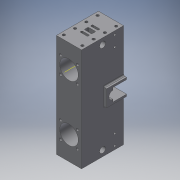
# Autodesk Inventor part: Carcassa
Saved by Autodesk Inventor 2016 (Build 200138000, 138)
## iProperties
Created: 2016-10-26
Part Number: Carcassa
Material: Generic
Document SubType Name: Modeling
Designer: 602199
Density: 1 g/cm^3
Appearance: Default
Author: 602199
Autodesk Inventor part; units mm, degrees
sketch "Sketch1" plane through (0, 0, 0) normal (0, 1, 0) x (-1, 0, 0)
  line L0 (-19, 77.75) -> (19, 77.75)
  line L1 (19, 77.75) -> (19, -77.75)
  line L2 (19, -77.75) -> (-19, -77.75)
  line L3 (-19, -77.75) -> (-19, 77.75)
  line L4 (-19, 77.75) -> (19, -77.75) construction
  line L5 (19, 77.75) -> (-19, -77.75) construction
  point P0 (0, 0)
  dimension "d0" = 38
  dimension "d1" = 155.5
  constraints: 12 end point, 2 midpoint, 2 parallel, 1 horizontal, 1 perpendicular
  measures "d0" distance of L1.end L2.end
  measures "d1" distance of L0.end L1.end
extrude "Extrusion1" add sketch "Sketch1" along normal blind 63.5
sketch "Sketch2" plane through (0, 0, 0) normal (1, 0, 0) x (0, 1, 0)
  line L0 (63.5, 77.75) -> (63.5, -77.75) construction
  line L1 (63.5, 0) -> (33.5, 0) construction
  line L2 (63.5, 0) -> (63.5, 12.5) construction
  line L3 (63.5, 12.5) -> (33.5, 12.5)
  line L4 (33.5, 12.5) -> (33.5, -12.5)
  line L5 (33.5, -12.5) -> (63.5, -12.5)
  line L6 (63.5, -12.5) -> (63.5, 12.5)
  point P0 (0, 0)
  dimension "d6" = 25
  constraints: 12 end point, 2 horizontal, 2 parallel, 1 midpoint, 1 perpendicular, 1 point on line
  measures "d6" distance of L4.end L3.end
extrude "Extrusion2" add sketch "Sketch2" along normal mid plane 47
sketch "Sketch3" plane through (0, 0, 0) normal (1, 0, 0) x (0, 1, 0)
  line L0 (63.5, 12.5) -> (63.5, -12.5) construction
  line L1 (63.5, 0) -> (42.8, 0) construction
  line L2 (63.5, 0) -> (63.5, 9.5) construction
  line L3 (63.5, 9.5) -> (42.8, 9.5)
  line L4 (42.8, 9.5) -> (42.8, -9.5)
  line L5 (42.8, -9.5) -> (63.5, -9.5)
  line L6 (63.5, -9.5) -> (63.5, 9.5)
  point P0 (0, 0)
  dimension "d9" = 20.7
  dimension "d11" = 9.5
  dimension "d12" = 19
  constraints: 12 end point, 2 horizontal, 2 parallel, 1 midpoint, 1 perpendicular, 1 point on line
  measures "d9" distance of L1.start L1.end
  measures "d11" distance of L1.start L2.end
  measures "d12" distance of L4.end L3.end
extrude "Extrusion3" cut sketch "Sketch3" along normal through all both and the other way through all
sketch "Sketch4" plane through (0, 0, 0) normal (1, 0, 0) x (0, 1, 0)
  line L0 (42.8, 9.5) -> (42.8, -9.5) projected
  circle A0 centre (42.8, 0) radius 6
  point P0 (0, 0)
  dimension "d15" = 12
  constraints: 1 centre point, 1 midpoint
  measures "d15" diameter of A0
extrude "Extrusion4" cut sketch "Sketch4" along normal through all both and the other way through all
sketch "Sketch5" plane through (19, 0, -77.75) normal (0, 0, -1) x (-1, 0, 0)
  line L0 (19, 0) -> (19, 63.5) construction
  line L1 (0, 63.5) -> (38, 63.5) construction
  line L2 (5, 6.25) -> (33, 6.25) construction
  line L3 (33, 6.25) -> (33, 57.25) construction
  line L4 (33, 57.25) -> (5, 57.25) construction
  line L5 (5, 57.25) -> (5, 6.25) construction
  line L6 (5, 6.25) -> (33, 57.25) construction
  line L7 (33, 6.25) -> (5, 57.25) construction
  circle A0 centre (5, 57.25) radius 2
  circle A1 centre (5, 6.25) radius 2
  circle A2 centre (33, 6.25) radius 2
  circle A3 centre (33, 57.25) radius 2
  line L8 (19, 31.75) -> (19, 40.25) construction
  line L9 (19, 40.25) -> (19, 23.25) construction
  circle A4 centre (5, 40.25) radius 2
  circle A5 centre (5, 23.25) radius 2
  circle A6 centre (33, 40.25) radius 2
  circle A7 centre (33, 23.25) radius 2
  dimension "d18" = 28
  dimension "d19" = 51
  dimension "d20" = 4
  dimension "d21" = 4
  dimension "d22" = 8.5
  dimension "d23" = 17
  constraints: 18 end point, 8 centre point, 6 point on line, 4 coincident, 4 midpoint, 2 parallel, 1 horizontal, 1 perpendicular
  measures "d18" distance of L4.end L3.end
  measures "d19" distance of L3.end L2.end
  measures "d20" diameter of A0
  measures "d21" diameter of A2
  measures "d22" distance of L8.start L8.end
  measures "d23" distance of L8.end L9.end
hole "Hole1" at (14, 57.25, -77.75) at (14, 40.25, -77.75) at (14, 23.25, -77.75) at (14, 6.25, -77.75) at (-14, 57.25, -77.75) at (-14, 40.25, -77.75) at (-14, 23.25, -77.75) at (-14, 6.25, -77.75) direction (0, 0, 1) diameter 4 depth 8
sketch "Sketch6" plane through (19, 0, -77.75) normal (0, 0, -1) x (-1, 0, 0)
  line L0 (19, 0) -> (19, 63.5) construction
  line L1 (0, 63.5) -> (38, 63.5) construction
  line L2 (5, 6.25) -> (33, 6.25) construction
  line L3 (33, 6.25) -> (33, 57.25) construction
  line L4 (33, 57.25) -> (5, 57.25) construction
  line L5 (5, 57.25) -> (5, 6.25) construction
  line L6 (5, 6.25) -> (33, 57.25) construction
  line L7 (33, 6.25) -> (5, 57.25) construction
  circle A0 centre (5, 57.25) radius 2
  circle A1 centre (5, 6.25) radius 2
  circle A2 centre (33, 6.25) radius 2
  circle A3 centre (33, 57.25) radius 2
  line L8 (19, 31.75) -> (19, 40.25) construction
  line L9 (19, 40.25) -> (19, 23.25) construction
  circle A4 centre (5, 40.25) radius 2
  circle A5 centre (5, 23.25) radius 2
  circle A6 centre (33, 40.25) radius 2
  circle A7 centre (33, 23.25) radius 2
  dimension "d31" = 28
  dimension "d32" = 51
  dimension "d33" = 4
  dimension "d34" = 4
  dimension "d35" = 8.5
  dimension "d36" = 17
  constraints: 20 end point, 8 centre point, 6 point on line, 4 coincident, 4 midpoint, 2 parallel, 1 horizontal, 1 perpendicular
  measures "d31" distance of L5.start L3.end
  measures "d32" distance of L3.end L3.start
  measures "d33" diameter of A0
  measures "d34" diameter of A2
  measures "d35" distance of L8.start L8.end
  measures "d36" distance of L8.end L9.end
hole "Hole2" at (14, 57.25, -77.75) at (-14, 57.25, -77.75) at (14, 40.25, -77.75) at (-14, 40.25, -77.75) at (-14, 23.25, -77.75) at (14, 23.25, -77.75) at (14, 6.25, -77.75) at (-14, 6.25, -77.75) direction (0, 0, 1) diameter 3.5 depth 12 tip angle 118
sketch "Sketch7" plane through (19, 0, -77.75) normal (0, 0, -1) x (-1, 0, 0)
  line L0 (0, 63.5) -> (38, 63.5) construction
  line L1 (19, 63.5) -> (19, 0) construction
  line L2 (19, 31.75) -> (38, 31.75) construction
  line L3 (13.25, 28.65) -> (24.75, 28.65)
  line L4 (24.75, 28.65) -> (24.75, 34.85)
  line L5 (24.75, 34.85) -> (13.25, 34.85)
  line L6 (13.25, 34.85) -> (13.25, 28.65)
  line L7 (13.25, 28.65) -> (24.75, 34.85) construction
  line L8 (24.75, 28.65) -> (13.25, 34.85) construction
  line L9 (19, 31.75) -> (19, 39.675) construction
  line L10 (19, 39.675) -> (19, 23.825) construction
  line L11 (13.25, 41.275) -> (24.75, 41.275)
  line L12 (24.75, 41.275) -> (24.75, 38.075)
  line L13 (24.75, 38.075) -> (13.25, 38.075)
  line L14 (13.25, 38.075) -> (13.25, 41.275)
  line L15 (13.25, 41.275) -> (24.75, 38.075) construction
  line L16 (24.75, 41.275) -> (13.25, 38.075) construction
  line L17 (13.25, 25.425) -> (24.75, 25.425)
  line L18 (24.75, 25.425) -> (24.75, 22.225)
  line L19 (24.75, 22.225) -> (13.25, 22.225)
  line L20 (13.25, 22.225) -> (13.25, 25.425)
  line L21 (13.25, 25.425) -> (24.75, 22.225) construction
  line L22 (24.75, 25.425) -> (13.25, 22.225) construction
  dimension "d44" = 11.5
  dimension "d45" = 6.2
  dimension "d46" = 7.925
  dimension "d47" = 15.85
  dimension "d48" = 11.5
  dimension "d49" = 3.2
  dimension "d50" = 3.2
  constraints: 44 end point, 8 midpoint, 6 parallel, 4 horizontal, 3 perpendicular, 3 point on line, 1 vertical
  measures "d44" distance of L5.end L4.end
  measures "d45" distance of L4.end L3.end
  measures "d46" distance of L2.start L9.end
  measures "d47" distance of L9.end L10.end
  measures "d48" distance of L12.end L13.end
  measures "d49" distance of L11.end L12.end
  measures "d50" distance of L17.end L18.end
extrude "Extrusion5" cut sketch "Sketch7" against normal blind 9
fillet "Fillet1" radius 1 12 edges at (5.75, 41.275, -73.25) (5.75, 38.075, -73.25) (5.75, 34.85, -73.25) (5.75, 28.65, -73.25) (5.75, 25.425, -73.25) (5.75, 22.225, -73.25) (-5.75, 22.225, -73.25) (-5.75, 25.425, -73.25) (-5.75, 34.85, -73.25) (-5.75, 28.65, -73.25) (-5.75, 38.075, -73.25) (-5.75, 41.275, -73.25)
sketch "Sketch8" plane through (19, 0, 77.75) normal (1, 0, 0) x (0, 0, -1)
  line L0 (155.5, 63.5) -> (133.5, 63.5) construction
  line L1 (90.25, 63.5) -> (155.5, 63.5) construction
  line L2 (133.5, 63.5) -> (133.5, 0) construction
  line L3 (155.5, 0) -> (0, 0) construction
  line L4 (155.5, 33.85) -> (155.5, 29.65) construction
  line L5 (155.5, 31.75) -> (151, 31.75) construction
  line L6 (155.5, 0) -> (142, 0) construction
  line L7 (142, 0) -> (142, 31.75) construction
  line L8 (142, 31.75) -> (151, 31.75) construction
  line L9 (146.5, 33.85) -> (146.5, 29.65) projected
  circle A0 centre (146.5, 31.75) radius 4.5
  point P0 (77.75, 0)
  dimension "d54" = 22
  dimension "d55" = 4.5
  dimension "d56" = 13.5
  constraints: 12 end point, 3 point on line, 2 midpoint, 2 perpendicular, 1 horizontal alignment, 1 vertical, 2 other
  measures "d54" distance of L0.start L0.end
  measures "d55" distance of L5.start L5.end
  measures "d56" distance of L3.start L6.end
extrude "Extrusion6" cut sketch "Sketch8" against normal blind 12
sketch "Sketch9" plane through (19, 0, 77.75) normal (1, 0, 0) x (0, 0, -1)
  line L0 (133.5, 63.5) -> (133.5, 0) construction
  line L1 (155.5, 33.85) -> (155.5, 29.65) construction
  line L2 (155.5, 31.75) -> (151, 31.75) construction
  line L3 (155.5, 0) -> (142, 0) construction
  line L4 (142, 0) -> (142, 31.75) construction
  line L5 (142, 31.75) -> (151, 31.75) construction
  line L6 (146.5, 33.85) -> (146.5, 29.65)
  circle A0 centre (146.5, 31.75) radius 4.5
  point P0 (77.75, 0)
  dimension "d60" = 4.5
  dimension "d61" = 13.5
  constraints: 14 end point, 2 midpoint, 2 perpendicular, 1 horizontal alignment, 1 vertical, 2 other
  measures "d60" distance of L2.start L2.end
  measures "d61" distance of L3.start L3.end
hole "Hole3" at (19, 31.75, -68.75) direction (-1, 0, 0) diameter 8.5 depth 22 tip angle 118
sketch "Sketch10" plane through (19, 0, 77.75) normal (1, 0, 0) x (0, 0, -1)
  arc A0 (71.75, 42.8) -> (83.75, 42.8) centre (77.75, 42.8) ccw construction
  line L0 (77.75, 42.8) -> (134.25, 42.8) construction
  line L1 (155.5, 63.5) -> (90.25, 63.5) construction
  line L2 (155.5, 63.5) -> (155.5, 50.3) construction
  line L3 (155.5, 0) -> (155.5, 63.5) construction
  line L4 (134.25, 63.5) -> (150.25, 63.5) construction
  line L5 (150.25, 63.5) -> (150.25, 50.3) construction
  circle A1 centre (150.25, 50.3) radius 1.5
  circle A2 centre (134.25, 50.3) radius 1.5
  point P0 (77.75, 0)
  dimension "d70" = 13.2
  dimension "d71" = 16
  dimension "d72" = 3
  constraints: 8 end point, 3 point on line, 2 centre point, 1 coincident, 1 horizontal, 1 perpendicular
  measures "d70" distance of L1.start L2.end
  measures "d71" distance of L4.start L4.end
  measures "d72" diameter of A1
extrude "Extrusion7" cut sketch "Sketch10" against normal blind 8
sketch "Sketch11" plane through (19, 0, 77.75) normal (1, 0, 0) x (0, 0, -1)
  line L0 (155.5, 63.5) -> (90.25, 63.5) construction
  line L1 (155.5, 63.5) -> (155.5, 50.3) construction
  line L2 (134.25, 63.5) -> (150.25, 63.5) construction
  line L3 (150.25, 63.5) -> (150.25, 50.3) construction
  circle A0 centre (150.25, 50.3) radius 1.4
  circle A1 centre (134.25, 50.3) radius 1.4
  point P0 (77.75, 0)
  point P1 (134.25, 42.8)
  dimension "d76" = 13.2
  dimension "d77" = 16
  dimension "d79" = 2.8
  dimension "d80" = 2.8
  constraints: 8 end point, 2 centre point, 2 point on line, 1 coincident, 1 perpendicular
  measures "d76" distance of L0.start L1.end
  measures "d77" distance of L2.start L2.end
  measures "d79" diameter of A0
  measures "d80" diameter of A1
hole "Hole4" at (19, 50.3, -56.5) at (19, 50.3, -72.5) direction (-1, 0, 0) diameter 2.8 depth 12 tip angle 118
ref_plane "Work Plane1" through (0, 0, 0) normal (0, 0, 1) x (1, 0, 0)
mirror "Mirror1" about plane through (0, 0, 0) normal (0, 0, 1) of "Hole4", "Extrusion7", "Hole3", "Extrusion6", "Fillet1", "Extrusion5", "Hole2", "Hole1"
sketch "Sketch14" plane through (0, 63.5, 0) normal (0, 1, 0) x (1, 0, 0)
  line L0 (0, 0) -> (0, 42.5) construction
  circle A0 centre (0, 42.5) radius 14
  line L1 (-16.3592, 0) -> (11.3099, 0) construction
  circle A1 centre (0, -42.5) radius 14
  dimension "d89" = 42.5
  dimension "d90" = 28
  constraints: 4 end point, 2 centre point, 1 coincident, 1 horizontal, 1 symmetric about line, 1 vertical, 1 other
  measures "d89" distance of L0.start L0.end
  measures "d90" diameter of A0
extrude "Extrusion8" cut sketch "Sketch14" against normal through all
sketch "Sketch15" plane through (0, 63.5, 0) normal (0, 1, 0) x (1, 0, 0)
  circle A0 centre (0, -42.5) radius 14 projected
  line L0 (0, -42.5) -> (0, -61.5)
  line L1 (7, -64.5) -> (-3, -64.5) projected
  line L2 (0, -61.5) -> (-5.5, -61.5)
  line L3 (-5.5, -61.5) -> (5.5, -61.5)
  line L4 (5.5, -61.5) -> (5.5, -50.5)
  line L5 (5.5, -50.5) -> (-5.5, -50.5)
  line L6 (-5.5, -50.5) -> (-5.5, -61.5)
  point P0 (0, 0)
  dimension "d94" = 19
  dimension "d95" = 5.5
  dimension "d96" = 11
  dimension "d97" = 11
  constraints: 12 end point, 3 perpendicular, 1 horizontal, 1 point on line, 1 vertical
  measures "d94" distance of L0.start L0.end
  measures "d95" distance of L0.end L2.end
  measures "d96" distance of L2.end L3.end
  measures "d97" distance of L3.end L4.end
extrude "Extrusion9" cut sketch "Sketch15" against normal blind 4.5 contours L6 L5 L0 A0 | A0 L0 L2 L6 | L4 L3 L0 A0 | A0 L0 L5 L4
sketch "Sketch16" plane through (0, 59, 0) normal (0, 1, 0) x (1, 0, 0)
  circle A0 centre (0, -42.5) radius 14 projected
  line L0 (0, -42.5) -> (0, -59.5)
  line L1 (0, -59.5) -> (-2, -59.5)
  line L2 (-2, -59.5) -> (2, -59.5)
  circle A1 centre (-2, -59.5) radius 1
  circle A2 centre (2, -59.5) radius 1
  point P0 (0, 0)
  dimension "d100" = 17
  dimension "d101" = 2
  dimension "d102" = 4
  dimension "d103" = 2
  dimension "d104" = 2
  constraints: 6 end point, 2 centre point, 2 coincident, 1 perpendicular, 1 point on line, 1 vertical
  measures "d100" distance of L0.start L0.end
  measures "d101" distance of L0.end L1.end
  measures "d102" distance of L1.end L2.end
  measures "d103" diameter of A1
  measures "d104" diameter of A2
hole "Hole5" at (-2, 59, 59.5) at (2, 59, 59.5) direction (0, -1, 0) diameter 2 depth 10 tip angle 118
sketch "Sketch17" plane through (0, 63.5, 0) normal (0, 1, 0) x (1, 0, 0)
  arc A0 (5.5, -55.3744) -> (-5.5, -55.3744) centre (0, -42.5) ccw projected
  circle A1 centre (0, -42.5) radius 18
  line L0 (0, -42.5) -> (12.7279, -29.7721)
  line L1 (0, -42.5) -> (18, -42.5) construction
  circle A2 centre (12.7279, -29.7721) radius 2
  point P0 (0, 0)
  dimension "d112" = 36
  dimension "d113" = 45
  dimension "d114" = 4
  constraints: 4 end point, 2 coincident, 1 centre point, 1 equal length, 1 horizontal, 3 other
  measures "d113" angle of L1 L0
  measures "d114" diameter of A2
hole "Hole6" at (12.7279, 63.5, 29.7721) direction (0, -1, 0) diameter 3.5 depth 20 tip angle 118 counterbore diameter 4 counterbore depth 8
pattern_circular "Circular Pattern1" count 4 over 360 about axis through (0, 63.5, 42.5) along (0, -1, 0) of "Hole6"
sketch "Sketch18" plane through (0, 63.5, 0) normal (0, 1, 0) x (1, 0, 0)
  line L0 (0, 0) -> (0, -13.79)
  line L1 (0, -13.79) -> (-13.79, -13.79)
  line L2 (0, -13.79) -> (13.79, -13.79)
  circle A0 centre (-13.79, -13.79) radius 2
  circle A1 centre (13.79, -13.79) radius 2
  dimension "d125" = 13.79
  dimension "d126" = 13.79
  dimension "d127" = 13.79
  dimension "d128" = 4
  dimension "d129" = 4
  constraints: 6 end point, 2 centre point, 2 coincident, 1 horizontal, 1 point on line, 1 vertical
  measures "d125" distance of L0.start L0.end
  measures "d126" distance of L0.end L1.end
  measures "d127" distance of L0.end L2.end
  measures "d128" diameter of A0
  measures "d129" diameter of A1
hole "Hole7" at (-13.79, 63.5, 13.79) at (13.79, 63.5, 13.79) direction (0, -1, 0) diameter 3.5 depth 20 tip angle 118 counterbore diameter 4 counterbore depth 8
ref_plane "Work Plane2" through (0, 0, 0) normal (0, 0, 1) x (1, 0, 0)
fillet "Fillet2" radius 2 2 edges at (-5.5, 61.25, 61.5) (5.5, 61.25, 61.5)
ref_plane "Work Plane3" through (0, 31.75, 0) normal (0, 1, 0) x (-1, 0, 0)
mirror "Mirror2" about plane through (0, 31.75, 0) normal (0, 1, 0) of "Hole6", "Circular Pattern1"
mirror "Mirror3" about plane through (0, 0, 0) normal (0, 0, 1) of "Hole6", "Hole5", "Extrusion9", "Circular Pattern1", "Hole7", "Fillet2", "Mirror2"
fillet "Fillet3" radius 2 4 edges at (19, 48.5, 12.5) (19, 48.5, -12.5) (-19, 48.5, -12.5) (-19, 48.5, 12.5)
body "Solid1"
